Autodesk Fusion 360 part; units mm, degrees
(part 2 of 2)
combine "Combine1" operation add target body 2 tool bodies 3 4 5 6 7 14 15 8 9 10 11 12 13 16 17 1 18 keep tools result as body 30 in component "bottom"
combine "Combine1'" operation add target body 20 tool bodies 21 22 23 24 25 26 27 28 29 19 keep tools result as body 31 in component "top-hipro"
extrude "Extrude1" [suppressed]
ref_plane "WorkPlane1" through (170, 56, 0.8) normal (0, 0, 1) x (1, 0, 0)
extrude "Extrude2" [suppressed]
ref_plane "WorkPlane2" through (170, 56, 4) normal (0, 0, 1) x (1, 0, 0)
extrude "Extrude3" [suppressed]
ref_plane "WorkPlane3" through (170, 56, 6.5) normal (0, 0, 1) x (1, 0, 0)
extrude "Extrude4" [suppressed]
extrude "Extrude5" [suppressed]
component "bottom" placed x (1, 0, 0) y (0, 1, 0) z (0, 0, 1) at (0, 0, 0)
component "top-hipro" placed x (1, 0, 0) y (0, 1, 0) z (0, 0, 1) at (0, 0, 0)
named bodies: "PCB", "b 2.0", "m b", "m t", "2.0"
